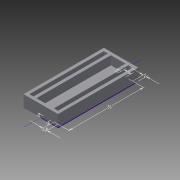
# Autodesk Inventor part: BasicConnector
Saved by Autodesk Inventor 2014 SP1 (Build 180222100, 222)
## iProperties
Created: 2015-03-29
Part Number: BasicConnector
Material: Generic
Document SubType Name: Modeling
Designer: Erin
Density: 1 g/cm^3
Appearance: Default
Author: Erin
Autodesk Inventor part; units mm, degrees
ref_plane "YZ Plane" through (0, 0, 0) normal (1, 0, 0) x (0, 1, 0)
ref_plane "XZ Plane" through (0, 0, 0) normal (0, 1, 0) x (-1, 0, 0)
ref_plane "XY Plane" through (0, 0, 0) normal (0, 0, 1) x (1, 0, 0)
sketch "Sketch1" plane through (0, 0, 0) normal (0, 0, 1) x (1, 0, 0)
  line L0 (0, 25.5) -> (5, 25.5)
  line L1 (5, 25.5) -> (5, -25.5)
  line L2 (5, -25.5) -> (0, -25.5)
  line L3 (0, -25.5) -> (0, 25.5)
  line L4 (5, 25.5) -> (7, 25.5)
  line L5 (7, 25.5) -> (7, -25.5)
  line L6 (7, -25.5) -> (5, -25.5)
  line L7 (5, -25.5) -> (5, 25.5)
  line L8 (7, 25.5) -> (9.8, 25.5)
  line L9 (9.8, 25.5) -> (9.8, -25.5)
  line L10 (9.8, -25.5) -> (7, -25.5)
  line L11 (7, -25.5) -> (7, 25.5)
  line L12 (9.8, -25.5) -> (11.8, -25.5)
  line L13 (11.8, -25.5) -> (11.8, 25.5)
  line L14 (11.8, 25.5) -> (9.8, 25.5)
  line L15 (9.8, 25.5) -> (9.8, -25.5)
  line L16 (0, 42.6516) -> (0, -39.217) construction
  line L17 (11.8, 25.5) -> (0, 25.5)
  line L18 (0, 25.5) -> (0, 27.5)
  line L19 (0, 27.5) -> (11.8, 27.5)
  line L20 (11.8, 27.5) -> (11.8, 25.5)
  line L21 (11.8, -25.5) -> (0, -25.5)
  line L22 (0, -25.5) -> (0, -27.5)
  line L23 (0, -27.5) -> (11.8, -27.5)
  line L24 (11.8, -27.5) -> (11.8, -25.5)
  point P0 (0, 0)
  point P1 (0, 0)
  dimension "d0" = 2
  dimension "d1" = 51
  dimension "d2" = 2.8
  dimension "d3" = 2
  dimension "d4" = 5
  dimension "d9" = 2
  dimension "d10" = 2
  constraints: 50 end point, 13 parallel, 6 horizontal, 6 perpendicular, 4 collinear, 2 point on line, 1 coincident, 1 midpoint, 1 vertical
  measures "d0" distance of L5.end L6.end
  measures "d1" distance of L4.end L5.end
  measures "d2" distance of L9.end L10.end
  measures "d3" distance of L14.end L13.end
  measures "d4" distance of L0.start L0.end
  measures "d9" distance of L17.end L18.end
  measures "d10" distance of L22.end L21.end
extrude "Extrusion1" add sketch "Sketch1" along normal blind 2 contours L0 L1 L2 L3 | L4 L5 L6 L1 | L8 L9 L10 L5 | L14 L13 L12 L9
extrude "Extrusion2" add sketch "Sketch1" along normal blind 8 contours L18 L19 L20 L14 L8 L4 L0 | L4 L5 L6 L1 | L2 L6 L10 L12 L24 L23 L22 | L14 L13 L12 L9
mirror "Mirror1" about plane through (0, 0, 0) normal (1, 0, 0) of "Extrusion1", "Extrusion2"
body "Solid1"
